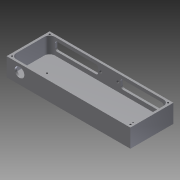
# Autodesk Inventor part: 13_1087_023
Saved by Autodesk Inventor 2014 SP1 (Build 180222100, 222)
## iProperties
Created: 2013-09-11
Part Number: 13_1087_023
Material: Allgemein
Document SubType Name: Modeling
Designer: vogel
Density: 1 g/cm^3
Appearance: Vorgabe
Author: vogel
Autodesk Inventor part; units mm, degrees
note: some values were not read from the file. Chosen so that the rebuilt part matches the saved one: direction of "Bohrung4".
ref_plane "YZ Plane" through (0, 0, 0) normal (1, 0, 0) x (0, 1, 0)
ref_plane "XZ Plane" through (0, 0, 0) normal (0, 1, 0) x (-1, 0, 0)
ref_plane "XY Plane" through (0, 0, 0) normal (0, 0, 1) x (1, 0, 0)
sketch "Skizze1" plane through (0, 0, 0) normal (0, 0, 1) x (1, 0, 0)
  line L0 (-23, 0) -> (138, 0) projected
  line L1 (0, -8) -> (0, 48) projected
  line L2 (0, 0) -> (115, 0)
  line L3 (115, 0) -> (115, 40)
  line L4 (115, 40) -> (0, 40)
  line L5 (0, 40) -> (0, 0)
  dimension "d0" = 40
  dimension "d1" = 115
  constraints: 8 end point, 2 parallel, 1 horizontal, 1 perpendicular
  measures "d0" distance of L4.end L2.start
  measures "d1" distance of L2.start L2.end
extrude "Extrusion1" add sketch "Skizze1" along normal blind 17
sketch "Skizze2" plane through (0, 0, 17) normal (0, 0, 1) x (1, 0, 0)
  line L0 (0, 0) -> (115, 0) projected
  line L1 (115, 0) -> (115, 40) projected
  line L2 (115, 40) -> (0, 40) projected
  line L3 (0, 40) -> (0, 0) projected
  line L4 (7, 38) -> (108, 38)
  line L5 (113, 33) -> (113, 7)
  line L6 (108, 2) -> (7, 2)
  line L7 (2, 7) -> (2, 33)
  arc A0 (7, 38) -> (2, 33) centre (7, 33) ccw
  arc A1 (113, 33) -> (108, 38) centre (108, 33) ccw
  arc A2 (108, 2) -> (113, 7) centre (108, 7) ccw
  arc A3 (2, 7) -> (7, 2) centre (7, 7) ccw
  dimension "d4" = 2
  dimension "d5" = 5
  constraints: 8 end point, 8 point on circle, 8 tangent, 4 centre point, 3 equal radius, 3 other
  measures "d4" distance between parallel lines of L4 L2
  measures "d5" radius of A0
extrude "Extrusion2" cut sketch "Skizze2" against normal blind 15 contours L4 A1 L5 A2 L6 A3 L7 A0
sketch "Skizze3" plane through (0, 0, 17) normal (0, 0, 1) x (1, 0, 0)
  line L0 (0, 0) -> (115, 0) projected
  line L1 (115, 0) -> (115, 40) projected
  line L2 (115, 40) -> (0, 40) projected
  line L3 (0, 40) -> (0, 0) projected
  line L4 (2.5, 37.5) -> (112.5, 37.5)
  line L5 (112.5, 37.5) -> (112.5, 2.5)
  line L6 (112.5, 2.5) -> (2.5, 2.5)
  line L7 (2.5, 2.5) -> (2.5, 37.5)
  dimension "d8" = 2.5
  constraints: 8 end point, 4 coincident, 3 other
  measures "d8" distance between parallel lines of L2 L4
hole "Bohrung1" at (112.5, 37.5, 17) at (112.5, 2.5, 17) at (2.5, 2.5, 17) at (2.5, 37.5, 17) direction (0, 0, -1) diameter 1.567 depth 6 tip angle 118 thread size "M2x0.4" class "6H" standard "ISO Metric profile"
sketch "Skizze4" plane through (0, 40, 0) normal (0, 1, 0) x (1, 0, 0)
  line L0 (0, 0) -> (0, -17) projected
  line L1 (113, -17) -> (108, -17) projected
  line L2 (113, -17) -> (108, -17) projected
  line L3 (113, -17) -> (113, -2) projected
  line L4 (113, -2) -> (108, -2) projected
  line L5 (108, -17) -> (108, -2) projected
  line L6 (108, -17) -> (7, -17) projected
  line L7 (108, -17) -> (108, -2) projected
  line L8 (108, -2) -> (7, -2) projected
  line L9 (7, -17) -> (7, -2) projected
  line L10 (88, -11) -> (88, -16) projected
  line L11 (108, -11) -> (88, -11) projected
  line L12 (108, -16) -> (108, -11) projected
  line L13 (88, -16) -> (108, -16) projected
  line L14 (-60.4, 0) -> (362.4, 0) projected
  line L15 (0, 3.4) -> (0, -20.4) projected
  arc A0 (118, -8) -> (118, -12) centre (118, -10) ccw projected
  line L16 (302, -14) -> (294, -14) projected
  line L17 (302, -6) -> (302, -14) projected
  line L18 (294, -6) -> (302, -6) projected
  line L19 (106, -14) -> (70, -14)
  line L20 (68, -12) -> (68, -8)
  line L21 (70, -6) -> (106, -6)
  line L22 (108, -8) -> (108, -12)
  arc A1 (108, -8) -> (106, -6) centre (106, -8) ccw
  arc A2 (106, -14) -> (108, -12) centre (106, -12) ccw
  arc A3 (68, -12) -> (70, -14) centre (70, -12) ccw
  arc A4 (70, -6) -> (68, -8) centre (70, -8) ccw
  line L23 (45, -14) -> (9, -14)
  line L24 (7, -12) -> (7, -8)
  line L25 (9, -6) -> (45, -6)
  line L26 (47, -8) -> (47, -12)
  arc A5 (45, -14) -> (47, -12) centre (45, -12) ccw
  arc A6 (47, -8) -> (45, -6) centre (45, -8) ccw
  arc A7 (9, -6) -> (7, -8) centre (9, -8) ccw
  arc A8 (7, -12) -> (9, -14) centre (9, -12) ccw
  line L27 (115, 0) -> (115, -17) projected
  arc A9 (283, -8) -> (281, -6) centre (281, -8) ccw projected
  line L28 (283, -8) -> (283, -12) projected
  arc A10 (281, -14) -> (283, -12) centre (281, -12) ccw projected
  line L29 (294, -14) -> (281, -14) projected
  line L30 (281, -6) -> (294, -6) projected
  point P0 (6, -6)
  point P1 (6, -14)
  point P2 (108, -14)
  point P3 (68, -6)
  point P4 (68, -14)
  point P5 (47, -14)
  point P6 (7, -6)
  dimension "d16" = 40
  dimension "d17" = 2
  dimension "d18" = 7
  dimension "d19" = 40
  dimension "d20" = 2
  dimension "d23" = 7
  constraints: 16 end point, 16 point on circle, 16 tangent, 11 point on line, 8 centre point, 6 equal radius, 4 parallel, 2 horizontal, 2 perpendicular, 1 other
  measures "d16" distance of point (108, -14) point (68, -14)
  measures "d17" radius of A1
  measures "d18" distance between parallel lines of L24 L0
  measures "d19" distance between parallel lines of L26 L24
  measures "d20" radius of A5
  measures "d23" distance between parallel lines of L5 L27
extrude "Extrusion3" cut sketch "Skizze4" against normal blind 2 contours A2 L19 L10 L11 L5 | L9 A7 L25 A6 L26 A5 L23 A8 | L5 L11 L10 L19 A3 L20 A4 L21 A1
sketch "Skizze5" plane through (0, 40, 0) normal (0, 1, 0) x (1, 0, 0)
  line L0 (0, 0) -> (0, -17) projected
  line L1 (115, -17) -> (0, -17) projected
  line L2 (115, 0) -> (115, -17) projected
  line L3 (0, -10) -> (115, -10)
  line L4 (115, 0) -> (0, 0) projected
  line L5 (57.5, -10) -> (57.5, -13.4142)
  point P0 (49.5, -10)
  point P1 (65.5, -10)
  dimension "d24" = 7
  dimension "d35" = 16
  constraints: 4 end point, 4 point on line, 2 perpendicular, 1 midpoint, 1 symmetric about line
  measures "d24" distance between parallel lines of L3 L1
  measures "d35" distance of point (65.5, -10) point (49.5, -10)
hole "Bohrung2" at (49.5, 40, 10) at (65.5, 40, 10) direction (0, -1, 0) diameter 2.459 depth 8 tip angle 118 thread size "M3x0.5" class "6H" standard "ISO Metric profile"
sketch "Skizze6" plane through (0, 0, 2) normal (0, 0, 1) x (1, 0, 0)
  line L0 (7, 38) -> (108, 38) projected
  line L1 (2, 7) -> (2, 33) projected
  line L2 (113, 33) -> (113, 7) projected
  line L3 (-23, 0) -> (138, 0) projected
  line L4 (0, -8) -> (0, 48) projected
  line L5 (2, 20) -> (113, 20)
  line L6 (57.5, 38) -> (57.5, 39.5212)
  point P0 (0, 0)
  point P1 (17.5, 20)
  point P2 (97.5, 20)
  dimension "d36" = 80
  constraints: 4 end point, 3 midpoint, 2 point on line, 1 perpendicular, 1 symmetric about line
  measures "d36" distance of point (97.5, 20) point (17.5, 20)
hole "Bohrung3" at (17.5, 20, 2) at (97.5, 20, 2) direction (0, 0, -1) diameter 1.567 end through all thread size "M2x0.4" class "6H" standard "ISO Metric profile"
sketch "Skizze7" plane through (0, 0, 0) normal (0, -1, 0) x (1, 0, 0)
  line L0 (0, 0) -> (115, 0) projected
  line L1 (0, 0) -> (0, 17) projected
  line L2 (0, 10) -> (20.9799, 10)
  line L3 (7, 17) -> (7, 2) projected
  point P0 (12, 10)
  dimension "d44" = 10
  dimension "d45" = 12
  constraints: 2 end point, 2 point on line, 1 perpendicular
  measures "d44" distance between parallel lines of L0 L2
  measures "d45" distance from line of L1 point (12, 10)
hole "Bohrung4" at (12, 0, 10) direction (0, 1, 0) diameter 9 end up to surface
